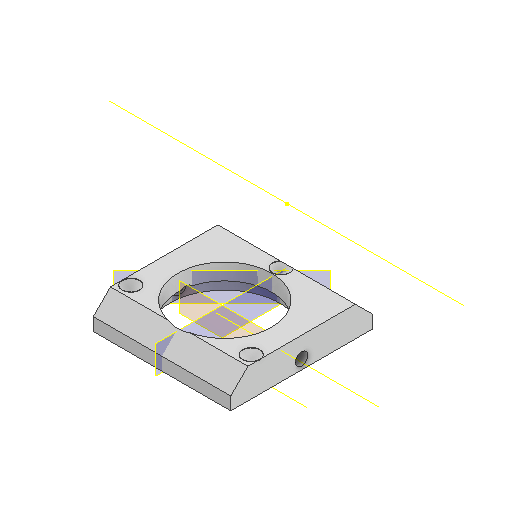
# Autodesk Inventor part: 20_Cube_Insert_Fibercombiner_FPC_filtermount_Thorlabs25mm_v3
Saved by Autodesk Inventor 2022 (Build 260153000, 153)
## iProperties
Created: 2021-12-04
Part Number: 20_Cube_Insert_Fibercombiner_FPC_filtermount_Thorlabs25mm_v3
Material: Generisch
Document SubType Name: Modeling
Designer: diederichbenedict
Density: 1 g/cm^3
Appearance: Vorgabe
Author: diederichbenedict
Autodesk Inventor part; units mm, degrees
ref_plane "YZ Plane" through (0, 0, 0) normal (1, 0, 0) x (0, 1, 0)
ref_plane "XZ Plane" through (0, 0, 0) normal (0, 1, 0) x (-1, 0, 0)
ref_plane "XY Plane" through (0, 0, 0) normal (0, 0, 1) x (1, 0, 0)
sketch "Skizze1" plane through (0, 0, 0) normal (0, 1, 0) x (-1, 0, 0)
  line L0 (0, 0) -> (-18, 0)
  line L1 (-18, 0) -> (-18, 28)
  line L2 (-18, 28) -> (0, 28)
  line L3 (0, 28) -> (0, 0)
  dimension "d0" = 18
  dimension "d1" = 28
  constraints: 8 end point, 2 parallel, 1 horizontal, 1 perpendicular
  measures "d0" distance of L1.end L2.end
  measures "d1" distance of L0.end L1.end
extrude "Extrusion1" add sketch "Skizze1" along normal blind 7
ref_plane "Arbeitsebene2" through (9, 0, 0) normal (-0.7071068, 0, -0.7071068) x (0, 1, 0)
ref_plane "Arbeitsebene1" through (9, 0, 0) normal (-1, 0, 0) x (0, 0, 1)
ref_plane "Arbeitsebene3" through (0, 0, 14) normal (0, 0, 1) x (1, 0, 0)
sketch "Skizze6" plane through (0, 0, 0) normal (-1, 0, 0) x (0, 0, 1)
  line L0 (0, 7) -> (28, 7) projected
  line L1 (0, 0) -> (0, 7) projected
  line L2 (0, 0) -> (28, 0) projected
  line L3 (28, 0) -> (28, 7) projected
  line L4 (0, 7) -> (-5, 7)
  line L5 (-5, 7) -> (-5, 0)
  line L6 (-5, 0) -> (0, 0)
  line L7 (0, 0) -> (0, 7)
  dimension "d24" = 5
  constraints: 8 end point, 2 parallel, 1 coincident, 1 horizontal, 1 perpendicular
  measures "d24" distance of L6.end L5.end
extrude "Extrusion6" add sketch "Skizze6" against normal up to surface (18 mm away) contours L1 L6 L5 L4
ref_plane "Arbeitsebene4" through (-15.85, 34.426, 14.0849) normal (0, 0.7071068, -0.7071068) x (1, 0, 0)
sketch "Skizze7" plane through (-15.85, 34.426, 14.0849) normal (0, 0.7071068, -0.7071068) x (1, 0, 0)
  point P0 (15.85, 34.3024)
sketch "Skizze8" plane through (0, 0, 0) normal (0, -1, 0) x (1, 0, 0)
  line L0 (0, 28) -> (18, 28) projected
  line L1 (18, 28) -> (18, -5) projected
  line L2 (0, -5) -> (0, 28) projected
  line L3 (0, -5) -> (-3, -5)
  line L4 (-3, -5) -> (-3, 28)
  line L5 (-3, 28) -> (0, 28)
  line L6 (0, 28) -> (0, -5)
  line L7 (18, 28) -> (18, -5) projected
  line L8 (18, 28) -> (21, 28)
  line L9 (21, 28) -> (21, -5)
  line L10 (21, -5) -> (18, -5)
  line L11 (18, -5) -> (18, 28)
  line L12 (0, -5) -> (0, 28) projected
  line L13 (0, -5) -> (18, -5) projected
  point P0 (0, 0)
  dimension "d27" = 3
  dimension "d28" = 3
  constraints: 16 end point, 4 parallel, 2 horizontal, 2 perpendicular, 1 point on line
  measures "d27" distance of L4.end L5.end
  measures "d28" distance of L9.end L10.end
extrude "Extrusion7" add sketch "Skizze8" against normal blind 7 contours L2 L3 L4 L5 | L8 L9 L10 L1
ref_plane "Arbeitsebene5" through (21, -5.7279, 12.7279) normal (0, 0.7071068, -0.7071068) x (-1, 0, 0)
sketch "Skizze10" plane through (-3, 0, -5) normal (-1, 0, 0) x (0, 0, 1)
  line L0 (0, 7) -> (33, 7) projected
  line L1 (0, 0) -> (0, 7) projected
  line L2 (33, 0) -> (0, 0) projected
  line L3 (33, 0) -> (33, 7) projected
  circle A0 centre (16.5, 2.2139) radius 1.45
  point P0 (5, 0)
  dimension "d38" = 2.9
  constraints: 1 centre point
  measures "d38" diameter of A0
extrude "Extrusion9" cut sketch "Skizze10" against normal through all contours A0
ref_plane "Arbeitsebene6" through (21, -1.4853, 8.4853) normal (0, 0.7071068, -0.7071068) x (-1, 0, 0)
sketch "Skizze15" plane through (21, 0, 28) normal (1, 0, 0) x (0, 0, -1)
  circle A0 centre (16.5, 2.2139) radius 1.45 projected
  line L0 (0, 7) -> (33, 7) projected
  line L1 (0, 0) -> (0, 7) projected
  line L2 (33, 0) -> (0, 0) projected
  line L3 (33, 0) -> (33, 7) projected
  line L4 (25.25, 7) -> (5, 7) projected
  line L5 (33.8464, 7) -> (33.8464, 0)
  point P0 (28, 0)
  point P1 (10.6096, 7)
  constraints: 2 end point, 2 point on line, 1 perpendicular
extrude "Extrusion10" add sketch "Skizze15" along normal blind 4
sketch "Skizze16" plane through (-3, 0, -5) normal (-1, 0, 0) x (0, 0, 1)
  line L0 (33, 7) -> (33, 0) projected
  line L1 (33, 0) -> (0, 0) projected
  line L2 (0, 7) -> (33, 7) projected
  line L3 (22.3904, 7) -> (0, 7)
  line L4 (0, 7) -> (0, 0)
  line L5 (0, 0) -> (22.3904, 0)
  line L6 (22.3904, 0) -> (22.3904, 7)
  line L7 (0, 0) -> (0, 7) projected
  circle A0 centre (16.5, 2.2139) radius 1.45 projected
  point P0 (5, 0)
  constraints: 8 end point, 2 parallel, 1 horizontal, 1 perpendicular
extrude "Extrusion11" add sketch "Skizze16" along normal blind 4
sketch "Skizze13" plane through (21, 7, 8.4853) normal (0, 1, 0) x (-1, 0, 0)
  circle A0 centre (-2, 12.7713) radius 2.45 projected
  circle A1 centre (26, 12.7713) radius 2.45 projected
  circle A2 centre (12, -8.2287) radius 2.75 projected
  point P0 (21, -4.9497)
  point P1 (12, -10.2287)
hole "Bohrung2" at (23, 7, 21.2566) at (-5, 7, 21.2566) at (9, 7, 0.2566) direction (0, -1, 0) diameter 4 depth 0.1 tip angle 118
chamfer "Fase3" distance 4 angle 45 2 edges at (9, 7, 28) (9, 7, -5)
sketch "Sketch17" plane through (0, 0, 0) normal (0, -1, 0) x (1, 0, 0)
  line L0 (25, 28) -> (25, -5) projected
  line L1 (-7, 28) -> (25, 28) projected
  line L2 (-7, -5) -> (-7, 28) projected
  circle A0 centre (9, 13.3904) radius 12.5 construction
  line L3 (-7, -5) -> (25, -5) projected
  circle A1 centre (9, 13.3904) radius 12.7 construction
  circle A2 centre (9, 13.3904) radius 12.8
  point P0 (0, 0)
  dimension "d70" = 25
  dimension "d75" = 0.1
  constraints: 2 centre point
  measures "d70" diameter of A0
  measures "d75" radial gap between concentric circles of A1 A2
extrude "Extrusion12" cut sketch "Sketch17" against normal blind 3.2 contours A2
sketch "Sketch18" plane through (0, 7, 0) normal (0, 1, 0) x (1, 0, 0)
  line L0 (-7, -28) -> (25, -28) projected
  line L1 (-7, 5) -> (-7, -28) projected
  line L2 (-7, 5) -> (25, 5) projected
  line L3 (25, -28) -> (25, 5) projected
  circle A0 centre (9, -13.3904) radius 10.8941
  point P0 (0, 0)
  constraints: 1 centre point
extrude "Extrusion13" cut sketch "Sketch18" against normal through all contours A0
